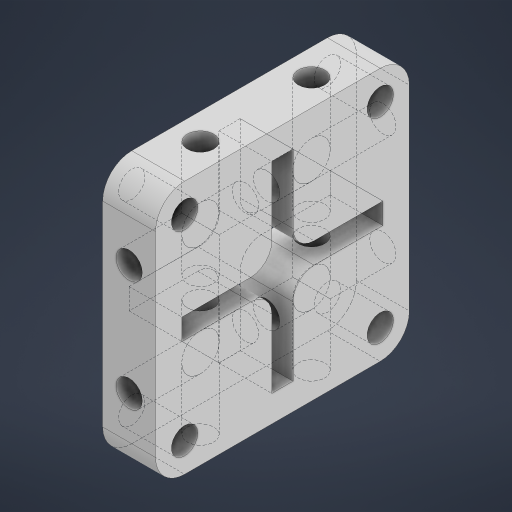
# Autodesk Inventor part: guidance_block
Saved by Autodesk Inventor 2024 (Build 280153000, 153)
## iProperties
Created: 2026-03-27
Part Number: guidance_block
Material: Generic
Document SubType Name: Modeling
Designer: schar
Density: 1 g/cm^3
Appearance: Default
Author: schar
Autodesk Inventor part; units mm, degrees
ref_plane "YZ Plane" through (0, 0, 0) normal (1, 0, 0) x (0, 1, 0)
ref_plane "XZ Plane" through (0, 0, 0) normal (0, 1, 0) x (-1, 0, 0)
ref_plane "XY Plane" through (0, 0, 0) normal (0, 0, 1) x (1, 0, 0)
sketch "Sketch1" plane through (0, 0, 0) normal (1, 0, 0) x (0, 1, 0)
  circle A0 centre (0, 0) radius 2.8284
  line L0 (0, 0) -> (-2.8284, 0)
  line L1 (-2.8284, 0) -> (-2.8284, -2.8284)
  line L2 (-2.8284, -2.8284) -> (0, -2.8284)
  line L3 (0, -2.8284) -> (0, 0)
  line L4 (0, 0) -> (-2.8284, -2.8284)
  line L5 (2, 2) -> (-2, 2)
  line L6 (-2, 2) -> (-2, -2)
  line L7 (-2, -2) -> (2, -2)
  line L8 (2, -2) -> (2, 2)
  line L9 (2, 2) -> (-2, -2) construction
  line L10 (-2, 2) -> (2, -2) construction
  line L11 (2, 2) -> (-2, 2)
  line L12 (-2, 2) -> (-2, 4)
  line L13 (-2, 4) -> (2, 4)
  line L14 (2, 4) -> (2, 2)
  line L15 (0, 4) -> (0, 19)
  line L16 (-2, 2) -> (-4, 2)
  line L17 (-4, 2) -> (-4, -2)
  line L18 (-4, -2) -> (-2, -2)
  line L19 (-4, 0) -> (-19, 0)
  line L20 (19, -19) -> (19, 19)
  line L21 (19, 19) -> (-19, 19)
  line L22 (-19, 19) -> (-19, -19)
  line L23 (-19, -19) -> (19, -19)
  line L24 (19, -19) -> (-19, 19) construction
  line L25 (19, 19) -> (-19, -19) construction
  line L26 (0, 19) -> (0, 24)
  line L27 (-19, 0) -> (-24, 0)
  line L28 (24, -24) -> (24, 24)
  line L29 (24, 24) -> (-24, 24)
  line L30 (-24, 24) -> (-24, -24)
  line L31 (-24, -24) -> (24, -24)
  line L32 (24, -24) -> (-24, 24) construction
  line L33 (24, 24) -> (-24, -24) construction
  line L34 (-2, 2) -> (-19, 2)
  line L35 (-19, -2) -> (-2, -2)
  line L36 (-2, -2) -> (-2, 2)
  line L37 (-2, -2) -> (-19, -2)
  line L38 (-19, -2) -> (-19, -19)
  line L39 (-19, -19) -> (-2, -19)
  line L40 (-2, -19) -> (-2, -2)
  line L41 (2, -2) -> (19, -2)
  line L42 (19, -2) -> (19, -19)
  line L43 (19, -19) -> (2, -19)
  line L44 (2, -19) -> (2, -2)
  line L45 (2, 2) -> (19, 2)
  line L46 (19, 2) -> (19, 19)
  line L47 (19, 19) -> (2, 19)
  line L48 (2, 19) -> (2, 2)
  line L49 (-2, 2) -> (-19, 2)
  line L50 (-19, 2) -> (-19, 19)
  line L51 (-19, 19) -> (-2, 19)
  line L52 (-2, 19) -> (-2, 2)
  point P0 (-2, 19)
  point P1 (2, 4)
  point P2 (2, -19)
  point P3 (-2, -19)
  dimension "d0" = 4
  dimension "d1" = 2
  dimension "d5" = 15
  dimension "d6" = 2
  dimension "d7" = 15
  dimension "d8" = 2
  dimension "d9" = 0
  dimension "d10" = 5
  dimension "d11" = 5
  dimension "d12" = 15
  dimension "d13" = 22.6716
  dimension "d14" = 20
  dimension "d15" = 29.7321
  constraints: 106 end point, 21 parallel, 12 perpendicular, 10 horizontal, 7 midpoint, 4 point on line, 2 coincident, 2 collinear, 2 point on circle, 2 tangent, 2 vertical, 1 centre point
  measures "d0" distance of L5.start L5.end
  measures "d1" distance of L11.end L12.end
  measures "d5" distance of L15.start L15.end
  measures "d6" distance of L11.end L16.end
  measures "d7" distance of L19.start L19.end
  measures "d8" distance from line of L16.end L19
  measures "d9" distance from line of L19.start L17
  measures "d10" distance of L15.end L26.end
  measures "d11" distance of L19.end L27.end
  measures "d12" distance between parallel lines of L21 L13
  measures "d13" distance of L20.end L13.end
  measures "d14" distance between parallel lines of L29 L13
  measures "d15" distance of L28.end L13.end
extrude "Extrusion1" add sketch "Sketch1" along normal blind 10 contours L14 L48 L21 L20 L45 | L41 L20 L23 L44 | L16 L34 L22 L21 L52 L12 | L20 L21 L26 L29 L28 L31 L30 L27 L22 L23 | L40 L2 L4 | L4 L1 L18 | L40 L23 L22 L35 L18 L1 L2 | L21 L22 L27 L30 L29 L26
sketch "Sketch2" plane through (0, 24, 24) normal (0, 1, 0) x (1, 0, 0)
  line L0 (10, 0) -> (0, 0) projected
  line L1 (0, 0) -> (0, 48) projected
  line L2 (0, 48) -> (10, 48) projected
  line L3 (10, 48) -> (10, 0) projected
  line L4 (0, 48) -> (10, 48) projected
  line L5 (0, 48) -> (0, 34.5)
  line L6 (0, 34.5) -> (5, 34.5)
  circle A0 centre (5, 34.5) radius 2.5
  line L7 (0, 0) -> (0, 13.5)
  line L8 (0, 22) -> (0, 5) projected
  line L9 (0, 13.5) -> (5, 13.5)
  circle A1 centre (5, 13.5) radius 2.5
  point P0 (0, 24)
  dimension "d18" = 13.5
  dimension "d19" = 5
  dimension "d20" = 5
  dimension "d21" = 13.5
  dimension "d22" = 5
  dimension "d23" = 5
  constraints: 8 end point, 2 centre point, 2 coincident, 2 perpendicular, 1 midpoint, 1 point on line
  measures "d18" distance of L1.end L5.end
  measures "d19" distance of L5.end L6.end
  measures "d20" diameter of A0
  measures "d21" distance of L0.end L7.end
  measures "d22" distance of L7.end L9.end
  measures "d23" diameter of A1
extrude "Extrusion2" cut sketch "Sketch2" against normal through all contours A0 | A1
sketch "Sketch3" plane through (0, -24, -24) normal (0, 0, -1) x (-1, 0, 0)
  line L0 (0, 0) -> (-10, 0) projected
  line L1 (0, 0) -> (0, 13.5)
  line L2 (0, 22) -> (0, 5) projected
  line L3 (0, 48) -> (-10, 48) projected
  line L4 (0, 48) -> (0, 34.5)
  line L5 (0, 0) -> (0, 48) projected
  line L6 (0, 34.5) -> (-5, 34.5)
  line L7 (0, 13.5) -> (-5, 13.5)
  circle A0 centre (-5, 13.5) radius 2.5
  circle A1 centre (-5, 34.5) radius 2.5
  point P0 (0, 24)
  dimension "d26" = 13.5
  dimension "d27" = 13.5
  dimension "d28" = 5
  dimension "d29" = 5
  dimension "d30" = 5
  dimension "d31" = 5
  constraints: 8 end point, 2 centre point, 2 coincident, 1 horizontal, 1 midpoint, 1 perpendicular, 1 point on line
  measures "d26" distance of L0.start L1.end
  measures "d27" distance of L3.start L4.end
  measures "d28" distance of L4.end L6.end
  measures "d29" distance of L1.end L7.end
  measures "d30" diameter of A0
  measures "d31" diameter of A1
extrude "Extrusion3" cut sketch "Sketch3" against normal through all
fillet "Fillet1" radius 4 4 edges at (5, -2, 2) (5, 2, 2) (5, 2, -2) (5, -2, -2)
sketch "Sketch4" plane through (10, 0, 0) normal (1, 0, 0) x (0, 0, -1)
  line L0 (24, 24) -> (-24, 24) projected
  line L1 (24, 24) -> (18.5, 24)
  line L2 (18.5, 24) -> (18.5, 18.5)
  line L3 (18.5, 18.5) -> (24, 18.5)
  line L4 (24, 18.5) -> (24, 24)
  circle A0 centre (18.5, 18.5) radius 2.5
  circle A1 centre (18.5, 18.5) radius 5.5
  circle A2 centre (-18.5, 18.5) radius 5.5
  circle A3 centre (-18.5, 18.5) radius 2.5
  line L5 (-18.5, 24) -> (-24, 24)
  line L6 (-24, 24) -> (-24, 18.5)
  circle A4 centre (-18.5, -18.5) radius 5.5
  circle A5 centre (-18.5, -18.5) radius 2.5
  line L7 (-24, -18.5) -> (-24, -24)
  line L8 (-24, -24) -> (-18.5, -24)
  circle A6 centre (18.5, -18.5) radius 5.5
  circle A7 centre (18.5, -18.5) radius 2.5
  line L9 (18.5, -24) -> (24, -24)
  line L10 (24, -24) -> (24, -18.5)
  point P0 (0, 0)
  point P1 (-18.5, 24)
  dimension "d35" = 5.5
  dimension "d36" = 5.5
  dimension "d37" = 5
  dimension "d40" = 360
  constraints: 20 end point, 5 coincident, 4 centre point, 2 parallel, 1 horizontal, 1 perpendicular, 49 other
  measures "d35" distance of L3.end L2.end
  measures "d36" distance of L2.end L1.end
  measures "d37" diameter of A0
extrude "Extrusion4" cut sketch "Sketch4" against normal through all contours L4 A1 L0 | A2 L6 L0 | A0 L3 L2 | L2 L3 A0 | A3 | A4 L8 L7 | A5 | L10 L9 A6 | A7
body "Solid1"
